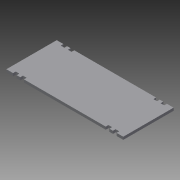
# Autodesk Inventor part: Oberteil
Saved by Autodesk Inventor 2015 (Build 190159000, 159)
## iProperties
Created: 2015-01-18
Part Number: Oberteil
Material: Generisch
Document SubType Name: Modeling
Designer: Jacob
Density: 1 g/cm^3
Appearance: Vorgabe
Author: Jacob
Autodesk Inventor part; units mm, degrees
ref_plane "YZ Plane" through (0, 0, 0) normal (1, 0, 0) x (0, 1, 0)
ref_plane "XZ Plane" through (0, 0, 0) normal (0, 1, 0) x (-1, 0, 0)
ref_plane "XY Plane" through (0, 0, 0) normal (0, 0, 1) x (1, 0, 0)
sketch "Skizze1" plane through (0, 0, 0) normal (0, 0, 1) x (1, 0, 0)
  line L0 (66.5, 29.5) -> (66.5, 1.5) projected
  line L1 (66.5, 1.5) -> (62.7599, 1.5) projected
  line L2 (62.7599, 1.5) -> (62.7599, 3) projected
  line L3 (62.7599, 3) -> (60.7599, 3) projected
  line L4 (60.7599, 3) -> (60.7599, 1.5) projected
  line L5 (60.7599, 1.5) -> (58.7599, 1.5) projected
  line L6 (58.7599, 1.5) -> (58.7599, 3) projected
  line L7 (58.7599, 3) -> (56.7599, 3) projected
  line L8 (56.7599, 3) -> (56.7599, 1.5) projected
  line L9 (56.7599, 1.5) -> (11.2401, 1.5) projected
  line L10 (11.2401, 1.5) -> (11.2401, 3) projected
  line L11 (11.2401, 3) -> (9.2401, 3) projected
  line L12 (9.2401, 3) -> (9.2401, 1.5) projected
  line L13 (9.2401, 1.5) -> (7.2401, 1.5) projected
  line L14 (7.2401, 1.5) -> (7.2401, 3) projected
  line L15 (7.2401, 3) -> (5.2401, 3) projected
  line L16 (5.2401, 3) -> (5.2401, 1.5) projected
  line L17 (5.2401, 1.5) -> (1.5, 1.5) projected
  line L18 (1.5, 1.5) -> (1.5, 29.5) projected
  line L19 (1.5, 29.5) -> (5.2401, 29.5) projected
  line L20 (5.2401, 29.5) -> (5.2401, 28) projected
  line L21 (5.2401, 28) -> (7.2401, 28) projected
  line L22 (7.2401, 28) -> (7.2401, 29.5) projected
  line L23 (7.2401, 29.5) -> (9.2401, 29.5) projected
  line L24 (9.2401, 29.5) -> (9.2401, 28) projected
  line L25 (9.2401, 28) -> (11.2401, 28) projected
  line L26 (11.2401, 28) -> (11.2401, 29.5) projected
  line L27 (11.2401, 29.5) -> (56.7599, 29.5) projected
  line L28 (56.7599, 29.5) -> (56.7599, 28) projected
  line L29 (56.7599, 28) -> (58.7599, 28) projected
  line L30 (58.7599, 28) -> (58.7599, 29.5) projected
  line L31 (58.7599, 29.5) -> (60.7599, 29.5) projected
  line L32 (60.7599, 29.5) -> (60.7599, 28) projected
  line L33 (60.7599, 28) -> (62.7599, 28) projected
  line L34 (62.7599, 28) -> (62.7599, 29.5) projected
  line L35 (62.7599, 29.5) -> (66.5, 29.5) projected
  line L36 (0, 0) -> (68, 0) projected
  line L37 (68, 0) -> (68, 31) projected
  line L38 (68, 31) -> (0, 31) projected
  line L39 (0, 31) -> (0, 0) projected
  line L40 (58.7599, 29.5) -> (58.7599, 28) projected
  line L41 (58.7599, 28) -> (56.7599, 28) projected
  line L42 (56.7599, 28) -> (56.7599, 29.5) projected
  line L43 (56.7599, 29.5) -> (11.2401, 29.5) projected
  line L44 (11.2401, 29.5) -> (11.2401, 28) projected
  line L45 (11.2401, 28) -> (9.2401, 28) projected
  line L46 (9.2401, 28) -> (9.2401, 29.5) projected
  line L47 (9.2401, 29.5) -> (7.2401, 29.5) projected
  line L48 (7.2401, 29.5) -> (7.2401, 28) projected
  line L49 (7.2401, 28) -> (5.2401, 28) projected
  line L50 (5.2401, 28) -> (5.2401, 29.5) projected
  line L51 (5.2401, 29.5) -> (1.5, 29.5) projected
  line L52 (1.5, 29.5) -> (1.5, 1.5) projected
  line L53 (1.5, 1.5) -> (5.2401, 1.5) projected
  line L54 (5.2401, 1.5) -> (5.2401, 3) projected
  line L55 (5.2401, 3) -> (7.2401, 3) projected
  line L56 (7.2401, 3) -> (7.2401, 1.5) projected
  line L57 (7.2401, 1.5) -> (9.2401, 1.5) projected
  line L58 (9.2401, 1.5) -> (9.2401, 3) projected
  line L59 (9.2401, 3) -> (11.2401, 3) projected
  line L60 (11.2401, 3) -> (11.2401, 1.5) projected
  line L61 (11.2401, 1.5) -> (56.7599, 1.5) projected
  line L62 (56.7599, 1.5) -> (56.7599, 3) projected
  line L63 (56.7599, 3) -> (58.7599, 3) projected
  line L64 (58.7599, 3) -> (58.7599, 1.5) projected
  line L65 (58.7599, 1.5) -> (60.7599, 1.5) projected
  line L66 (60.7599, 1.5) -> (60.7599, 3) projected
  line L67 (60.7599, 3) -> (62.7599, 3) projected
  line L68 (62.7599, 3) -> (62.7599, 1.5) projected
  line L69 (62.7599, 1.5) -> (66.5, 1.5) projected
  line L70 (66.5, 1.5) -> (66.5, 29.5) projected
  line L71 (66.5, 29.5) -> (62.7599, 29.5) projected
  line L72 (62.7599, 29.5) -> (62.7599, 28) projected
  line L73 (62.7599, 28) -> (60.7599, 28) projected
  line L74 (60.7599, 28) -> (60.7599, 29.5) projected
  line L75 (60.7599, 29.5) -> (58.7599, 29.5) projected
  line L76 (58.7599, 29.5) -> (58.7599, 28) projected
  line L77 (58.7599, 28) -> (56.7599, 28) projected
  line L78 (56.7599, 28) -> (56.7599, 29.5) projected
  line L79 (56.7599, 29.5) -> (11.2401, 29.5) projected
  line L80 (11.2401, 29.5) -> (11.2401, 28) projected
  line L81 (11.2401, 28) -> (9.2401, 28) projected
  line L82 (9.2401, 28) -> (9.2401, 29.5) projected
  line L83 (9.2401, 29.5) -> (7.2401, 29.5) projected
  line L84 (7.2401, 29.5) -> (7.2401, 28) projected
  line L85 (7.2401, 28) -> (5.2401, 28) projected
  line L86 (5.2401, 28) -> (5.2401, 29.5) projected
  line L87 (5.2401, 29.5) -> (1.5, 29.5) projected
  line L88 (1.5, 29.5) -> (1.5, 1.5) projected
  line L89 (1.5, 1.5) -> (5.2401, 1.5) projected
  line L90 (5.2401, 1.5) -> (5.2401, 3) projected
  line L91 (5.2401, 3) -> (7.2401, 3) projected
  line L92 (7.2401, 3) -> (7.2401, 1.5) projected
  line L93 (7.2401, 1.5) -> (9.2401, 1.5) projected
  line L94 (9.2401, 1.5) -> (9.2401, 3) projected
  line L95 (9.2401, 3) -> (11.2401, 3) projected
  line L96 (11.2401, 3) -> (11.2401, 1.5) projected
  line L97 (11.2401, 1.5) -> (56.7599, 1.5) projected
  line L98 (56.7599, 1.5) -> (56.7599, 3) projected
  line L99 (56.7599, 3) -> (58.7599, 3) projected
  line L100 (58.7599, 3) -> (58.7599, 1.5) projected
  line L101 (58.7599, 1.5) -> (60.7599, 1.5) projected
  line L102 (60.7599, 1.5) -> (60.7599, 3) projected
  line L103 (60.7599, 3) -> (62.7599, 3) projected
  line L104 (62.7599, 3) -> (62.7599, 1.5) projected
  line L105 (62.7599, 1.5) -> (66.5, 1.5) projected
  line L106 (66.5, 1.5) -> (66.5, 29.5) projected
  line L107 (66.5, 29.5) -> (62.7599, 29.5) projected
  line L108 (62.7599, 29.5) -> (62.7599, 28) projected
  line L109 (62.7599, 28) -> (60.7599, 28) projected
  line L110 (60.7599, 28) -> (60.7599, 29.5) projected
  line L111 (60.7599, 29.5) -> (58.7599, 29.5) projected
  line L112 (1.5, 1.5) -> (66.5, 1.5)
  line L113 (66.5, 1.5) -> (66.5, 29.5)
  line L114 (66.5, 29.5) -> (1.5, 29.5)
  line L115 (1.5, 29.5) -> (1.5, 1.5)
  line L116 (0, 0) -> (68, 0)
  line L117 (68, 0) -> (68, 31)
  line L118 (68, 31) -> (0, 31)
  line L119 (0, 31) -> (0, 0)
  constraints: 16 end point, 4 parallel, 2 horizontal, 2 perpendicular
extrude "Extrusion1" add sketch "Skizze1" along normal blind 1.5 contours L0 L1 L2 L3 L4 L5 L6 L7 L8 L9 L10 L11 L12 L13 L14 L15 L16 L17 L18 L19 L20 L21 L22 L23 L24 L25 L26 L27 L28 L29 L30 L31 L32 L33 L34 L35
